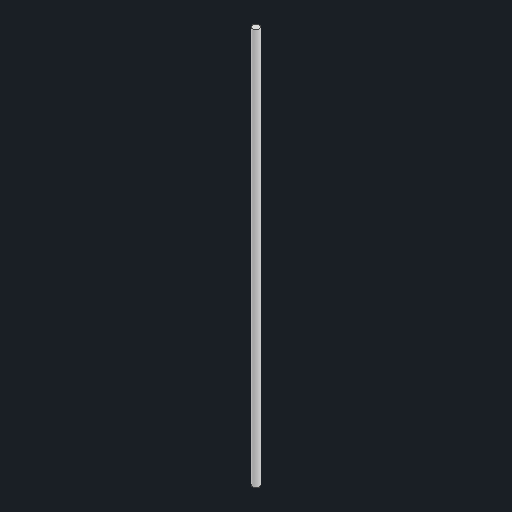
# Autodesk Inventor part: S05
Saved by Autodesk Inventor 2027 (Build 310192000, 192)
## iProperties
Created: 2026-04-27
Part Number: S05
Material: Generic
Description: #5 BAR X (SCHEDULED LENGTH)
Document SubType Name: Modeling
Designer: mstri
Density: 1 g/cm^3
Appearance: Default
MCP_RevitFamily: S05
MCP_RevitElemIds: 4628940,4628941
MANUFACTURE_COMPONENT: REBAR CUSTOM ASSEMBLY COMPONENT RAW CONSUMABLE
CONTROL_MARK: STRAIGHT BAR
SORTING_ORDER: 520
IDENTITY_DESCRIPTION_SHORT: S05
IDENTITY_DESCRIPTION: #5 BAR X (SCHEDULED LENGTH)
DIM_LENGTH: 3
QTY_MULTIPLIER: 1
ASSEMBLY_COMPONENT: 1
BAR_TYPE_CIP: 0
BAR_TYPE_EMBED: 0
BAR_TYPE_ERECTION: 0
BAR_TYPE_ENDREINFORCING: 0
BAR_TYPE_STRIPPING: 0
MCP_REVIT_SOURCE_ELEMENT_ID: 4628940
Author: mstri
Autodesk Inventor part; units mm, degrees
ref_plane "YZ Plane" through (0, 0, 0) normal (1, 0, 0) x (0, 1, 0)
ref_plane "XZ Plane" through (0, 0, 0) normal (0, 1, 0) x (-1, 0, 0)
ref_plane "XY Plane" through (0, 0, 0) normal (0, 0, 1) x (1, 0, 0)
sketch "S05_Profile" plane through (0, 0, 0) normal (0, 1, 0) x (-1, 0, 0)
  circle A0 centre (0, 0) radius 7.9375
  constraints: 1 centre point
extrude "S05_BarBody" add sketch "S05_Profile" along normal blind 914.4
equation "\"BarLength\" = 914.4"
equation "\"BarDiameter\" = 15.875"
equation "\"DIM_LENGTH\" = 914.4"
body "Solid3"
